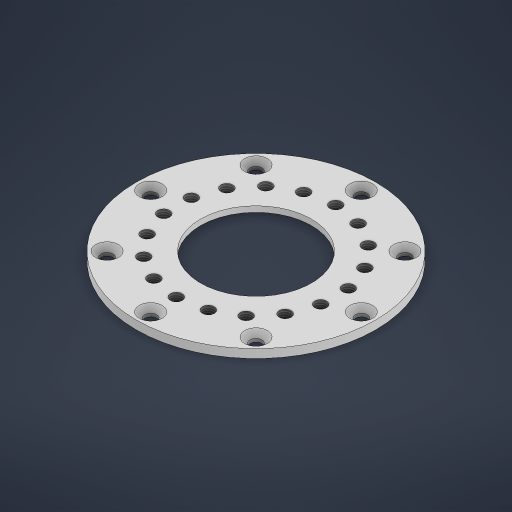
# Autodesk Inventor part: HousingLid
Saved by Autodesk Inventor 2024 (Build 280153000, 153)
## iProperties
Created: 2024-02-01
Part Number: HousingLid
Material: Generic
Document SubType Name: Modeling
Designer: avsar
Density: 1 g/cm^3
Appearance: Default
Author: avsar
Autodesk Inventor part; units mm, degrees
ref_plane "YZ Plane" through (0, 0, 0) normal (1, 0, 0) x (0, 1, 0)
ref_plane "XZ Plane" through (0, 0, 0) normal (0, 1, 0) x (-1, 0, 0)
ref_plane "XY Plane" through (0, 0, 0) normal (0, 0, 1) x (1, 0, 0)
sketch "Sketch1" plane through (0, 0, 0) normal (0, 1, 0) x (-1, 0, 0)
  circle A0 centre (0, 0) radius 42
  circle A1 centre (0, 0) radius 19.5
  circle A2 centre (0, -37) radius 2.1
  circle A3 centre (26.163, -26.163) radius 2.1
  circle A4 centre (37, 0) radius 2.1
  circle A5 centre (26.163, 26.163) radius 2.1
  circle A6 centre (0, 37) radius 2.1
  circle A7 centre (-26.163, 26.163) radius 2.1
  circle A8 centre (-37, 0) radius 2.1
  circle A9 centre (-26.163, -26.163) radius 2.1
  dimension "d0" = 84
  dimension "d1" = 39
  dimension "d2" = 4.2
  dimension "d3" = 37
  dimension "d6" = 360
  constraints: 10 centre point, 2 coincident, 1 vertical alignment, 17 other
  measures "d0" diameter of A0
  measures "d1" diameter of A1
  measures "d2" diameter of A2
  measures "d3" distance of A2.centre point (0, 0)
extrude "Extrusion1" add sketch "Sketch1" against normal blind 3
sketch "Sketch2" plane through (0, -3, 0) normal (0, -1, 0) x (1, 0, 0)
  circle A0 centre (0, 0) radius 24
  dimension "d10" = 48
  constraints: 1 centre point, 1 coincident
  measures "d10" diameter of A0
extrude "Extrusion2" cut sketch "Sketch2" against normal blind 1
hole "Hole1" at (37, 0, 0) at (26.163, 0, 26.163) at (0, 0, 37) at (-26.163, 0, 26.163) at (-37, 0, 0) at (-26.163, 0, -26.163) at (0, 0, -37) at (26.163, 0, -26.163) direction (0, -1, 0) diameter 4.2 end through all countersink diameter 8 countersink angle 90
sketch "Sketch3" plane through (0, 0, 0) normal (0, 1, 0) x (1, 0, 0)
  circle A0 centre (0, -28) radius 2.1
  circle A1 centre (9.5766, -26.3114) radius 2.1
  circle A2 centre (17.9981, -21.4492) radius 2.1
  circle A3 centre (24.2487, -14) radius 2.1
  circle A4 centre (27.5746, -4.8621) radius 2.1
  circle A5 centre (27.5746, 4.8621) radius 2.1
  circle A6 centre (24.2487, 14) radius 2.1
  circle A7 centre (17.9981, 21.4492) radius 2.1
  circle A8 centre (9.5766, 26.3114) radius 2.1
  circle A9 centre (0, 28) radius 2.1
  circle A10 centre (-9.5766, 26.3114) radius 2.1
  circle A11 centre (-17.9981, 21.4492) radius 2.1
  circle A12 centre (-24.2487, 14) radius 2.1
  circle A13 centre (-27.5746, 4.8621) radius 2.1
  circle A14 centre (-27.5746, -4.8621) radius 2.1
  circle A15 centre (-24.2487, -14) radius 2.1
  circle A16 centre (-17.9981, -21.4492) radius 2.1
  circle A17 centre (-9.5766, -26.3114) radius 2.1
  point P0 (0, 0)
  dimension "d20" = 4.2
  dimension "d21" = 28
  dimension "d24" = 360
  constraints: 18 centre point, 1 vertical alignment, 37 other
  measures "d20" diameter of A0
  measures "d21" distance of point (0, 0) A0.centre
extrude "Extrusion3" cut sketch "Sketch3" against normal through all
thread "Thread1" size "M4.5x0.75" class "6H" standard "ANSI Metric M Profile" full length
thread "Thread2" size "M4.5x0.75" class "6H" standard "ANSI Metric M Profile" full length
thread "Thread3" size "M4.5x0.75" class "6H" standard "ANSI Metric M Profile" full length
thread "Thread4" size "M4.5x0.75" class "6H" standard "ANSI Metric M Profile" full length
thread "Thread5" size "M4.5x0.75" class "6H" standard "ANSI Metric M Profile" full length
thread "Thread6" size "M4.5x0.75" class "6H" standard "ANSI Metric M Profile" full length
thread "Thread7" size "M4.5x0.75" class "6H" standard "ANSI Metric M Profile" full length
thread "Thread8" size "M4.5x0.75" class "6H" standard "ANSI Metric M Profile" full length
thread "Thread9" size "M4.5x0.75" class "6H" standard "ANSI Metric M Profile" full length
thread "Thread10" size "M4.5x0.75" class "6H" standard "ANSI Metric M Profile" full length
thread "Thread11" size "M4.5x0.75" class "6H" standard "ANSI Metric M Profile" full length
thread "Thread12" size "M4.5x0.75" class "6H" standard "ANSI Metric M Profile" full length
thread "Thread13" size "M4.5x0.75" class "6H" standard "ANSI Metric M Profile" full length
thread "Thread14" size "M4.5x0.75" class "6H" standard "ANSI Metric M Profile" full length
thread "Thread15" size "M4.5x0.75" class "6H" standard "ANSI Metric M Profile" full length
thread "Thread16" size "M4.5x0.75" class "6H" standard "ANSI Metric M Profile" full length
thread "Thread17" size "M4.5x0.75" class "6H" standard "ANSI Metric M Profile" full length
thread "Thread18" size "M4.5x0.75" class "6H" standard "ANSI Metric M Profile" full length
body "Solid1"
